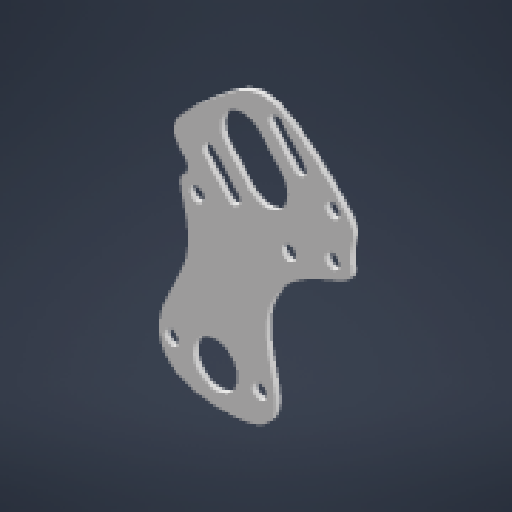
# Autodesk Inventor part: third-stage
Saved by Autodesk Inventor 2023 (Build 270158000, 158)
## iProperties
Created: 2023-03-29
Part Number: third-stage
Material: Generic
Document SubType Name: Modeling
Designer: Liam
Density: 1 g/cm^3
Appearance: Default
Author: Liam
Autodesk Inventor part; units mm, degrees
ref_plane "YZ Plane" through (0, 0, 0) normal (1, 0, 0) x (0, 1, 0)
ref_plane "XZ Plane" through (0, 0, 0) normal (0, 1, 0) x (-1, 0, 0)
ref_plane "XY Plane" through (0, 0, 0) normal (0, 0, 1) x (1, 0, 0)
sketch "Sketch1" plane through (0, 0, 0) normal (0, 0, 1) x (1, 0, 0)
  line L0 (-72.8164, 47.6422) -> (-79.5151, 55.2811)
  line L1 (-63.5697, 69.2654) -> (-56.8709, 61.6266)
  circle A0 centre (-45.6184, 44.45) radius 2.0955
  circle A1 centre (-45.6184, 57.15) radius 2.0955
  line L2 (-78.2217, 69.8899) -> (-79.1765, 69.0525)
  line L3 (-78.2217, 69.8899) -> (-77.2668, 70.7272)
  line L4 (-60.0895, 58.8441) -> (-66.7486, 66.4377)
  line L5 (-69.638, 50.4706) -> (-76.2972, 58.0643)
  line L6 (-53.7199, 64.3898) -> (-60.4186, 72.0287)
  line L7 (-75.9674, 44.879) -> (-82.6661, 52.5179)
  arc A2 (-75.9674, 44.879) -> (-72.8164, 47.6422) centre (-74.3919, 46.2606) ccw
  arc A3 (-79.5151, 55.2811) -> (-82.6661, 52.5179) centre (-81.0906, 53.8995) ccw
  arc A4 (-56.8709, 61.6266) -> (-53.7199, 64.3898) centre (-55.2954, 63.0082) ccw
  arc A5 (-60.4186, 72.0287) -> (-63.5697, 69.2654) centre (-61.9942, 70.647) ccw
  arc A6 (-69.638, 50.4706) -> (-60.0895, 58.8441) centre (-64.8638, 54.6573) ccw
  arc A7 (-66.7486, 66.4377) -> (-76.2972, 58.0643) centre (-71.5229, 62.251) ccw
  line L8 (-82.6661, 52.5179) -> (-79.5151, 55.2811) construction
  line L9 (-76.2972, 58.0643) -> (-66.7486, 66.4377) construction
  line L10 (-63.5697, 69.2654) -> (-60.4186, 72.0287) construction
  circle A8 centre (-79.3648, 1.8096) radius 6.35
  line L11 (-88.5156, 44.9984) -> (-91.6915, 42.3545) construction
  line L12 (-91.6915, 42.3545) -> (-81.0906, 27.4698) construction
  line L13 (-81.0906, 27.4698) -> (-97.6874, 11.6223) construction
  line L14 (-97.6874, 11.6223) -> (-96.3761, -5.5105) construction
  line L15 (-96.3761, -5.5105) -> (-83.114, -9.5834) construction
  line L16 (-83.114, -9.5834) -> (-50.7251, -8.7363) construction
  line L17 (-50.7251, -8.7363) -> (-70.3989, 17.9685) construction
  line L18 (-70.3989, 17.9685) -> (-63.5612, 33.0418) construction
  line L19 (-63.5612, 33.0418) -> (-56.8709, 37.4727) construction
  spline S0 degree 4 poles (-88.5156, 44.9984) (-91.6915, 42.3545) (-81.0906, 27.4698) (-97.6874, 11.6223) (-96.3761, -5.5105) (-83.114, -9.5834) (-50.7251, -8.7363) (-70.3989, 17.9685) (-63.5612, 33.0418) (-56.8709, 37.4727) knots 1 1 1 1 1 2 3 4 5 6 7 7 7 7 7
  line L20 (-88.5156, 44.9984) -> (-85.3396, 47.6422) construction
  line L21 (-85.3396, 47.6422) -> (-93.4914, 52.5179) construction
  line L22 (-93.4914, 52.5179) -> (-92.1298, 57.6933) construction
  line L23 (-92.1298, 57.6933) -> (-79.1765, 69.0525) construction
  line L24 (-79.1765, 69.0525) -> (-68.1262, 77.6396) construction
  line L25 (-68.1262, 77.6396) -> (-58.947, 75.2527) construction
  line L26 (-58.947, 75.2527) -> (-39.2684, 57.015) construction
  line L27 (-39.2684, 57.015) -> (-39.2684, 53.4754) construction
  line L28 (-39.2684, 53.4754) -> (-41.525, 48.2396) construction
  line L29 (-41.525, 48.2396) -> (-39.2044, 42.3545) construction
  line L30 (-39.2044, 42.3545) -> (-41.9553, 40.9734) construction
  line L31 (-41.9553, 40.9734) -> (-50.1806, 41.9035) construction
  line L32 (-50.1806, 41.9035) -> (-56.8709, 37.4727) construction
  spline S1 degree 4 poles (-88.5156, 44.9984) (-85.3396, 47.6422) (-93.4914, 52.5179) (-92.1298, 57.6933) (-79.1765, 69.0525) (-68.1262, 77.6396) (-58.947, 75.2527) (-39.2684, 57.015) (-39.2684, 53.4754) (-41.525, 48.2396) (-39.2044, 42.3545) (-41.9553, 40.9734) (-50.1806, 41.9035) (-56.8709, 37.4727) knots 1 1 1 1 1 2 3 4 5 6 7 8 9 10 11 11 11 11 11
  circle A9 centre (-58.2829, 40.2547) radius 2.0955
  circle A10 centre (-84.7892, 41.664) radius 2.0955
  circle A11 centre (-66.6703, 1.4359) radius 2.0955
  circle A12 centre (-92.0593, 2.1834) radius 2.0955
  line L33 (-92.0593, 2.1834) -> (-79.3648, 1.8096) construction
  line L34 (-79.3648, 1.8096) -> (-66.6703, 1.4359) construction
  circle A13 centre (-71.4316, 20.7646) radius 2.0955
  circle A14 centre (-82.2396, 29.27) radius 2.0955
  point P0 (0, 0)
  point P1 (-79.3931, 52.0233)
  point P2 (-61.9743, 70.6245)
  point P3 (-81.0715, 53.8776)
  point P4 (-71.5229, 62.251)
  point P5 (-81.0906, 53.8995)
  dimension "d18" = 1.27
  dimension "d22" = 1.27
  dimension "d23" = 4.191
  dimension "d24" = 4.191
  dimension "d42" = 10.16
  dimension "d43" = 10.16
  dimension "d47" = 4.191
  dimension "d48" = 4.191
  dimension "d51" = 6.35
  dimension "d52" = 6.35
  dimension "d54" = 12.7
  dimension "d55" = 12.7
  dimension "d56" = 12.7
  dimension "d57" = 12.7
  dimension "d60" = 4.191
  dimension "d61" = 4.191
  dimension "d62" = 12.7
  dimension "d63" = 4.191
  dimension "d64" = 4.191
  dimension "d65" = 12.7
  dimension "d68" = 4.191
  dimension "d69" = 4.191
  constraints: 26 end point, 15 centre point, 12 point on circle, 9 tangent, 6 equal length, 5 parallel, 4 collinear, 3 midpoint, 2 perpendicular, 2 point on line, 1 coincident, 1 vertical, 9 other
  measures "d18" distance of L2.start L2.end
  measures "d22" distance of L2.start L3.end
  measures "d23" diameter of A0
  measures "d24" diameter of A1
  measures "d42" distance of L0.start L0.end
  measures "d43" distance of L1.start L1.end
  measures "d47" distance between parallel lines of L0 L7
  measures "d48" distance between parallel lines of L6 L1
  measures "d51" radius of A6
  measures "d52" radius of A7
  measures "d54" distance of point (-71.523, 62.251) point (-61.994, 70.647)
  measures "d55" distance of point (-81.091, 53.899) A7.centre
  measures "d56" distance of A6.centre A4.centre
  measures "d57" distance of A2.centre A6.centre
  measures "d60" diameter of A9
  measures "d61" diameter of A10
  measures "d62" diameter of A8
  measures "d63" diameter of A11
  measures "d64" diameter of A12
  measures "d65" distance of L33.end L33.start
  measures "d68" diameter of A13
  measures "d69" diameter of A14
extrude "Extrusion4" add sketch "Sketch1" along normal blind 1.524
body "Solid4"
